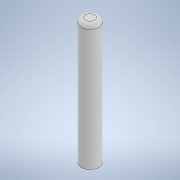
# Autodesk Inventor part: fixture_pi_guide_pin
Saved by Autodesk Inventor 2022 (Build 260153000, 153)
## iProperties
Created: 2022-02-17
Part Number: fixture_pi_guide_pin
Material: Generic
Document SubType Name: Modeling
Designer: Thomas
Density: 1 g/cm^3
Appearance: Default
Author: Thomas
Autodesk Inventor part; units mm, degrees
ref_plane "YZ Plane" through (0, 0, 0) normal (1, 0, 0) x (0, 1, 0)
ref_plane "XZ Plane" through (0, 0, 0) normal (0, 1, 0) x (-1, 0, 0)
ref_plane "XY Plane" through (0, 0, 0) normal (0, 0, 1) x (1, 0, 0)
sketch "Sketch1" plane through (0, 0, 0) normal (0, 1, 0) x (-1, 0, 0)
  circle A0 centre (0, 0) radius 1.05
  dimension "d0" = 2.1
  constraints: 1 centre point, 1 coincident
  measures "d0" diameter of A0
extrude "Extrusion1" add sketch "Sketch1" along normal blind 15
fillet "Fillet1" radius 0.5 1 edges at (1.05, 15, 0)
body "Solid1"
